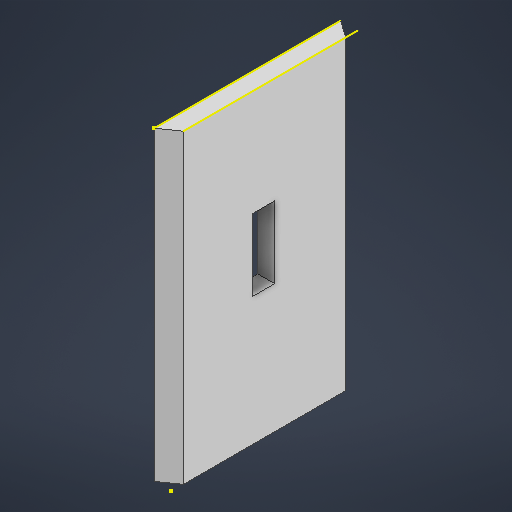
# Autodesk Inventor part: Part2
Saved by Autodesk Inventor 2026.1 (Build 301233000, 233)
## iProperties
Created: 2025-08-25
Part Number: Part2
Material: Generic
Document SubType Name: Modeling
Designer: usman
Density: 1 g/cm^3
Appearance: Default
Author: usman
Autodesk Inventor part; units mm, degrees
ref_plane "YZ Plane" through (0, 0, 0) normal (1, 0, 0) x (0, 1, 0)
ref_plane "XZ Plane" through (0, 0, 0) normal (0, 1, 0) x (-1, 0, 0)
ref_plane "XY Plane" through (0, 0, 0) normal (0, 0, 1) x (1, 0, 0)
sketch "Sketch1" plane through (0, 0, 0) normal (1, 0, 0) x (0, 1, 0)
  line L0 (0, 0) -> (179, 0)
  line L1 (179, 0) -> (179, -109)
  line L2 (179, -109) -> (0, -109)
  line L3 (0, -109) -> (0, 0)
  dimension "d0" = 179
  dimension "d1" = 109
  constraints: 8 end point, 2 parallel, 1 horizontal, 1 perpendicular
  measures "d0" distance of L1.end L2.end
  measures "d1" distance of L0.end L1.end
extrude "Extrusion1" add sketch "Sketch1" along normal blind 10
sketch "Sketch2" plane through (0, 179, 0) normal (0, 1, 0) x (1, 0, 0)
  point P0 (0, 0)
sketch "Sketch3" plane through (0, 179, 0) normal (0, 1, 0) x (1, 0, 0)
  line L0 (0, 109) -> (10, 101.9979)
  line L1 (10, 109) -> (10, 0) projected
  line L2 (0, 109) -> (0, 0) projected
  line L3 (0, 0) -> (10, 0) projected
  line L4 (0, 0) -> (10, 7.0021)
  dimension "d4" = 125
  dimension "d5" = 125
  constraints: 4 end point, 2 point on line
  measures "d4" angle of L2 L0
  measures "d5" angle of L2 L4
extrude "Extrusion2" cut sketch "Sketch3" against normal through all contours L4 L1 L3
sketch "Sketch4" plane through (0, 179, -109) normal (0, 1, 0) x (1, 0, 0)
  point P0 (0, -109)
sketch "Sketch5" plane through (0, 179, -109) normal (0, 1, 0) x (1, 0, 0)
  line L0 (0, -109) -> (0, 0) projected
  line L1 (10, 0) -> (10, -101.9979) projected
sketch "Sketch6" plane through (0, 179, -109) normal (0, 1, 0) x (1, 0, 0)
  line L0 (0, -109) -> (0, 0) projected
  line L1 (0, 0) -> (10, -7.0021)
  line L2 (10, 0) -> (10, -101.9979) projected
  line L3 (0, 0) -> (10, 0)
  line L4 (0, 0) -> (10, 0) projected
  line L5 (10, 0) -> (10, -7.0021)
  dimension "d8" = 125
  constraints: 6 end point, 1 collinear, 1 perpendicular, 1 point on line
  measures "d8" angle of L2 L1
extrude "Extrusion3" cut sketch "Sketch6" against normal through all
sketch "Sketch7" plane through (10, 0, 0) normal (1, 0, 0) x (0, 0, -1)
  point P0 (0, 0)
sketch "Sketch8" plane through (10, 0, 0) normal (1, 0, 0) x (0, 0, -1)
  line L0 (47.4589, 117) -> (60.4589, 117)
  line L1 (60.4589, 117) -> (60.4589, 75)
  line L2 (60.4589, 75) -> (47.4589, 75)
  line L3 (47.4589, 75) -> (47.4589, 117)
  line L4 (101.9979, 179) -> (7.0021, 179) projected
  point P0 (0, 0)
  dimension "d11" = 13
  dimension "d12" = 42
  dimension "d13" = 62
  constraints: 8 end point, 2 parallel, 1 horizontal, 1 perpendicular
  measures "d11" distance of L0.start L0.end
  measures "d12" distance of L0.end L1.end
  measures "d13" distance between parallel lines of L0 L4
extrude "Extrusion4" cut sketch "Sketch8" against normal through all
body "Solid1"
